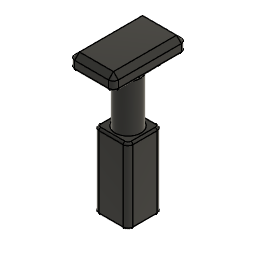
Buffer (Autodesk Fusion 360 design; units mm, degrees)
Autodesk Fusion 360 part; units mm, degrees
note: some values were not read from the file. Chosen so that the rebuilt part matches the saved one: which bodies a step acts on. Set by a fixed rule: which sketch regions a step uses.
sketch "Sketch1" plane through (0, 0, 0) normal (0, 0, 1) x (1, 0, 0)
  line L0 (3.5, -3.5) -> (-3.5, -3.5)
  line L1 (-3.5, -3.5) -> (-3.5, 3.5)
  line L2 (-3.5, 3.5) -> (3.5, 3.5)
  line L3 (3.5, 3.5) -> (3.5, -3.5)
  line L4 (3.5, -3.5) -> (-3.5, 3.5) construction
  line L5 (-3.5, -3.5) -> (3.5, 3.5) construction
  dimension "d1" = 7
  dimension "d2" = 7
  constraint horizontal L0
  constraint perpendicular L0 L1
  constraint parallel L0 L2
  constraint parallel L1 L3
  constraint coincident L4 origin
  constraint coincident L5 origin
  measures "d1" distance of L1.end L2.end
  measures "d2" distance of L0.end L1.end
extrude "Extrude1" add sketch "Sketch1" along normal blind 15.5 makes body 1
sketch "Sketch2" plane through (0, 0, 15.5) normal (0, 0, 1) x (-1, 0, 0)
  line L0 (-3.5, -3.5) -> (3.5, -3.5)
  line L1 (3.5, -3.5) -> (3.5, 3.5)
  line L2 (3.5, 3.5) -> (-3.5, 3.5)
  line L3 (-3.5, 3.5) -> (-3.5, -3.5)
  circle A0 centre (0, 0) radius 2.5
  dimension "d5" = 5
  constraint coincident A0.centre origin
  measures "d5" diameter of A0
extrude "Extrude2" add sketch "Sketch2" along normal blind 6 contours A0 bodies 1
sketch "Sketch3" plane through (0, 0, 21.5) normal (0, 0, 1) x (-1, 0, 0)
  circle A0 centre (0, 0) radius 2.5
  line L0 (-4.5, -7.5) -> (4.5, -7.5)
  line L1 (4.5, -7.5) -> (4.5, 7.5)
  line L2 (4.5, 7.5) -> (-4.5, 7.5)
  line L3 (-4.5, 7.5) -> (-4.5, -7.5)
  line L4 (-4.5, -7.5) -> (4.5, 7.5) construction
  line L5 (4.5, -7.5) -> (-4.5, 7.5) construction
  dimension "d8" = 9
  dimension "d9" = 15
  constraint horizontal L0
  constraint perpendicular L0 L1
  constraint parallel L0 L2
  constraint parallel L1 L3
  constraint coincident L4 A0.centre
  constraint coincident L5 A0.centre
  constraint coincident A0.centre origin
  measures "d8" distance of L1.end L2.end
  measures "d9" distance of L0.end L1.end
extrude "Extrude3" add sketch "Sketch3" along normal blind 3 contours A0 | L0 L1 L2 L3 bodies 1
fillet "Fillet1" radius 1 4 edges at (4.5, 7.5, 23) (4.5, -7.5, 23) (-4.5, -7.5, 23) (-4.5, 7.5, 23) on bodies 1
chamfer "Chamfer2" distance 1 distance2 1 1 faces at (1.5, -2.1667, 24.5) on bodies 1
fillet "Fillet2" radius 2 1 edges at (2.3308, 0.904, 21.5) on bodies 1
fillet "Fillet3" radius 0.5 8 edges at (4.5, 0, 21.5) (4.2071, 7.2071, 21.5) (0, 7.5, 21.5) (-4.2071, 7.2071, 21.5) (-4.5, 0, 21.5) (-4.2071, -7.2071, 21.5) (0, -7.5, 21.5) (4.2071, -7.2071, 21.5) on bodies 1
fillet "Fillet3" radius 1 4 edges at (3.5, -3.5, 7.75) (-3.5, -3.5, 7.75) (3.5, 3.5, 7.75) (-3.5, 3.5, 7.75) on bodies 1
sketch "Sketch4" plane through (0, 0, 15.5) normal (0, 0, 1) x (-1, 0, 0)
  arc A0 (2.5, -3.5) -> (3.5, -2.5) centre (2.5, -2.5) ccw
  line L0 (3.5, -2.5) -> (3.5, 2.5)
  arc A1 (3.5, 2.5) -> (2.5, 3.5) centre (2.5, 2.5) ccw
  line L1 (2.5, 3.5) -> (-2.5, 3.5)
  arc A2 (-2.5, 3.5) -> (-3.5, 2.5) centre (-2.5, 2.5) ccw
  line L2 (-3.5, 2.5) -> (-3.5, -2.5)
  arc A3 (-3.5, -2.5) -> (-2.5, -3.5) centre (-2.5, -2.5) ccw
  line L3 (-2.5, -3.5) -> (2.5, -3.5)
  circle A4 centre (0, 0) radius 2.5
  circle A5 centre (0, 0) radius 2.5
  circle A6 centre (0, 0) radius 2.8
  dimension "d24" = 0.3
extrude "Extrude4" cut sketch "Sketch4" against normal blind 12 contours A4 A5 | A6 bodies 1 makes body 2 at (1.1667, -2.1667, 24.5)
extrude "Extrude5" add 1 faces at (0.8863, -0.2321, 15.5) along direction (0, 0, -1) blind 6 on bodies 2 bodies 2
coil "CoilPrimitive1" add diameter 4 section square size 1 on centre turns 3 pitch 5 right hand placed x (-1, 0, 0) y (0, -1, 0) z (0, 0, 1) at (0, 0, 3.5) separate body makes body 3
sketch "Sketch5" plane through (0, 0, 15.5) normal (0, 0, 1) x (-1, 0, 0)
  circle A0 centre (0, 0) radius 2.8
  arc A1 (2.5, -3.5) -> (3.5, -2.5) centre (2.5, -2.5) ccw
  line L0 (3.5, -2.5) -> (3.5, 2.5)
  arc A2 (3.5, 2.5) -> (2.5, 3.5) centre (2.5, 2.5) ccw
  line L1 (2.5, 3.5) -> (-2.5, 3.5)
  arc A3 (-2.5, 3.5) -> (-3.5, 2.5) centre (-2.5, 2.5) ccw
  line L2 (-3.5, 2.5) -> (-3.5, -2.5)
  arc A4 (-3.5, -2.5) -> (-2.5, -3.5) centre (-2.5, -2.5) ccw
  line L3 (-2.5, -3.5) -> (2.5, -3.5)
  circle A5 centre (0, 0) radius 2.65
  dimension "d34" = 5.3
  constraint concentric A0 A5
  measures "d34" diameter of A5
extrude "Extrude6" add sketch "Sketch5" against normal blind 5 contours A0 bodies 1
chamfer "Chamfer3" distance 0.15 distance2 0.15 1 edges at (2.6105, 1.0125, 10.5) measured on face at (-2.7861, 0.2788, 8.1667) on bodies 1
sketch "Sketch6" plane through (0, 0, 9.5) normal (0, 0, -1) x (1, 0, 0)
  circle A0 centre (0, 0) radius 2.5
  circle A1 centre (0, 0) radius 2.65
  dimension "d39" = 5.3
  constraint concentric A0 A1
  measures "d39" diameter of A1
extrude "Extrude7" add sketch "Sketch6" against normal blind 1 bodies 2
chamfer "Chamfer4" distance 0.15 distance2 0.15 1 edges at (2.3308, 0.904, 10.5) measured on face at (-2.4876, -0.2489, 13.5) on bodies 2
move_body "Move1" bodies 3 to x (1, 0, 0) y (0, 1, 0) z (0, 0, 1) at (0, 0, -2.5)
extrude "Extrude9" cut 1 faces at (0.5487, 0.2642, 3.5) along direction (0, 0, -1) blind 2 on bodies 1 bodies 1
sketch "Sketch7" plane through (0, 0, 15.5) normal (0, 0, 1) x (-1, 0, 0)
  circle A0 centre (0, 0) radius 2.65
  arc A1 (2.5, -3.5) -> (3.5, -2.5) centre (2.5, -2.5) ccw
  line L0 (3.5, -2.5) -> (3.5, 2.5)
  arc A2 (3.5, 2.5) -> (2.5, 3.5) centre (2.5, 2.5) ccw
  line L1 (2.5, 3.5) -> (-2.5, 3.5)
  arc A3 (-2.5, 3.5) -> (-3.5, 2.5) centre (-2.5, 2.5) ccw
  line L2 (-3.5, 2.5) -> (-3.5, -2.5)
  arc A4 (-3.5, -2.5) -> (-2.5, -3.5) centre (-2.5, -2.5) ccw
  line L3 (-2.5, -3.5) -> (2.5, -3.5)
  line L4 (2.5812, 0.6) -> (3.5, 0.6)
  line L5 (2.5812, -0.6) -> (3.5, -0.6)
  line L6 (2.65, 0) -> (3.5, 0)
  line L7 (3.5, 0.6) -> (3.5, -0.6)
  line L8 (3.0406, 0.6) -> (3.0406, -0.6)
  dimension "d44" = 0.6
  dimension "d45" = 0.6
  constraint coincident A0 L4.start
  constraint coincident L0 L4.end
  constraint perpendicular L0 L4
  constraint coincident A0 L5.start
  constraint coincident L0 L5.end
  constraint perpendicular L0 L5
  constraint coincident A0 L6.start
  constraint midpoint L0 L6.end
  constraint perpendicular L0 L6
  constraint midpoint L4 L8.start
  constraint midpoint L5 L8.end
  measures "d44" distance of L4 L6
  measures "d45" distance of L5 L6
extrude "Extrude8" cut sketch "Sketch7" against normal blind 14 contours A0 L5 L6 L8 | A0 L4 L6 L8 bodies 1
sketch "Sketch8" plane through (0, 0, 9.5) normal (0, 0, -1) x (1, 0, 0)
  circle A0 centre (0, 0) radius 2.65
  circle A1 centre (0, 0) radius 2.5
  line L0 (-2.4495, 0.5) -> (-2.9495, 0.5)
  line L1 (-2.9495, 0.5) -> (-2.9495, -0.5)
  line L2 (-2.9495, -0.5) -> (-2.4495, -0.5)
  line L3 (-2.5, 0) -> (-3.2, 0)
  dimension "d50" = 5
  dimension "d51" = 0.5
  dimension "d52" = 0.5
  dimension "d53" = 0.5
  dimension "d59" = 0.7
  constraint concentric A0 A1
  constraint coincident A1 L0.start
  constraint horizontal L0
  constraint perpendicular L0 L1
  constraint coincident A1 L2.end
  constraint perpendicular L1 L2
  constraint coincident A1 L3.start
  constraint horizontal L3
  measures "d50" diameter of A1
  measures "d51" distance of L0 L3
  measures "d52" distance of L2 L3
  measures "d53" distance of L0.start L0.end
  measures "d59" distance of L3.start L3.end
extrude "Extrude10" add sketch "Sketch8" against normal blind 9 contours A0 A1 L0 L3 | A0 L0 L1 L3 | A0 L1 L2 L3 | A0 A1 L2 L3 bodies 2
chamfer "Chamfer5" distance 0.45 angle 45 1 edges at (-2.5, 0, 18.5) on bodies 2
extrude "Extrude11" add 1 faces at (-0.0428, 0.7627, 1.5) along direction (0, 0, 1) blind 0.5 on bodies 1 bodies 1 3
extrude "Extrude12" cut 1 faces at (0.5367, -0.2603, 9.5) along direction (0, 0, 1) blind 1.15 on bodies 2 bodies 2
extrude "Extrude13" add 1 faces at (-0.3932, 0.6228, 10.65) along direction (0, 0, -1) blind 4.5 on bodies 2 bodies 2
sketch "Sketch9" plane through (0, 0, 6.15) normal (0, 0, -1) x (1, 0, 0)
  line L0 (-2.9495, -0.5) -> (-2.4495, -0.5)
  arc A0 (-2.4495, -0.5) -> (-2.4495, 0.5) centre (0, 0) ccw
  line L1 (-2.4495, 0.5) -> (-2.9495, 0.5)
  line L2 (-2.9495, 0.5) -> (-2.9495, -0.5)
  circle A1 centre (0, 0) radius 2.65
  dimension "d64" = 5.3
  constraint concentric A0 A1
  measures "d64" diameter of A1
extrude "Extrude14" add sketch "Sketch9" along normal blind 1.15 bodies 2
chamfer "Chamfer6" distance 0.15 angle 45 1 edges at (2.5, 0, 6.15) on bodies 2
move_body "Move3" bodies 2 to x (1, 0, 0) y (0, 1, 0) z (0, 0, 1) at (0, 0, 5.65)
fillet "Fillet4" radius 0.4 17 edges at (3.2071, -3.2071, 15.5) (0, -3.5, 15.5) (-3.2071, -3.2071, 15.5) (-3.5, 0, 15.5) (-3.2071, 3.2071, 15.5) (0, 3.5, 15.5) (3.2071, 3.2071, 15.5) (3.5, 0, 15.5) (0, -3.5, 0) (-3.2071, -3.2071, 0) (-3.5, 0, 0) (-3.2071, 3.2071, 0) (0, 3.5, 0) (3.2071, 3.2071, 0) (3.5, 0, 0) (3.2071, -3.2071, 0) (2.65, 0, 10.65) on bodies 1 2
fillet "Fillet5" radius 0.4 1 edges at (-2.9495, 0, 10.65) on bodies 2
equation "d45 = d44"
equation "d64 = ( 2.65 * 2 ) * 1 mm"
named bodies: "Holder", "Buffer"
